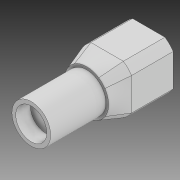
# Autodesk Inventor part: J0_Post
Saved by Autodesk Inventor 2020 (Build 240168000, 168)
## iProperties
Created: 2021-06-12
Part Number: J0_Post
Material: Generic
Document SubType Name: Modeling
Designer: DDeGo
Density: 1 g/cm^3
Appearance: Default
Author: DDeGo
Autodesk Inventor part; units mm, degrees
ref_plane "YZ Plane" through (0, 0, 0) normal (1, 0, 0) x (0, 1, 0)
ref_plane "XZ Plane" through (0, 0, 0) normal (0, 1, 0) x (-1, 0, 0)
sketch "Sketch1" plane through (0, 0, 0) normal (0, 0, 1) x (1, 0, 0)
  circle A0 centre (0, 0) radius 6
  dimension "d0" = 12
  constraints: 1 centre point, 1 coincident
  measures "d0" diameter of A0
extrude "Extrusion1" add sketch "Sketch1" along normal blind 24
sketch "Sketch2" plane through (0, 0, 0) normal (0, 0, -1) x (-1, 0, 0)
  line L0 (-5, -5) -> (5, -5)
  line L1 (5, -5) -> (5, 5)
  line L2 (5, 5) -> (-5, 5)
  line L3 (-5, 5) -> (-5, -5)
  line L4 (-5, -5) -> (5, 5) construction
  line L5 (5, -5) -> (-5, 5) construction
  circle A0 centre (0, 0) radius 7.723
  dimension "d3" = 10
  dimension "d4" = 10
  constraints: 12 end point, 2 midpoint, 2 parallel, 1 centre point, 1 coincident, 1 horizontal, 1 perpendicular
  measures "d3" distance of L1.end L2.end
  measures "d4" distance of L0.end L1.end
extrude "Extrusion2" cut sketch "Sketch2" against normal blind 8.5
sketch "Sketch3" plane through (0, 0, 24) normal (0, 0, 1) x (1, 0, 0)
  circle A0 centre (0, 0) radius 3.175
  dimension "d7" = 6.35
  constraints: 1 centre point, 1 coincident
  measures "d7" diameter of A0
extrude "Extrusion3" cut sketch "Sketch3" against normal blind 3
ref_plane "Work Plane1" through (0, 0, 12.7) normal (0, 0, -1) x (-1, 0, 0)
sketch "Sketch5" plane through (0, 0, 24) normal (0, 0, 1) x (1, 0, 0)
  circle A0 centre (0, 0) radius 3.96
  circle A1 centre (0, 0) radius 11.6408
  dimension "d14" = 7.92
  constraints: 2 centre point, 2 coincident
  measures "d14" diameter of A0
extrude "Extrusion4" cut sketch "Sketch5" against normal up to surface (15.5 mm away)
sketch "Sketch6" plane through (-3.3166, 5, 8.5) normal (0, 0, 1) x (1, 0, 0)
  line L0 (8.3166, -1.6834) -> (8.3166, -8.3166) projected
  arc A0 (8.3166, -1.6834) -> (6.6332, 0) centre (3.3166, -5) ccw projected
  line L1 (0, 0) -> (6.6332, 0) projected
  arc A1 (0, 0) -> (-1.6834, -1.6834) centre (3.3166, -5) ccw projected
  line L2 (-1.6834, -8.3166) -> (-1.6834, -1.6834) projected
  arc A2 (-1.6834, -8.3166) -> (0, -10) centre (3.3166, -5) ccw projected
  line L3 (6.6332, -10) -> (0, -10) projected
  arc A3 (6.6332, -10) -> (8.3166, -8.3166) centre (3.3166, -5) ccw projected
  circle A4 centre (3.3166, -5) radius 3.96 construction
sketch "Sketch7" plane through (0, 0, 12.7) normal (0, 0, -1) x (-1, 0, 0)
  circle A0 centre (0, 0) radius 3.96 construction
  circle A1 centre (0, 0) radius 3.175 construction
  circle A2 centre (0, 0) radius 4.5
  dimension "d18" = 9
  constraints: 1 centre point, 1 coincident
  measures "d18" diameter of A2
loft "Loft1" add profiles "Sketch6", "Sketch7"
body "Solid1"
